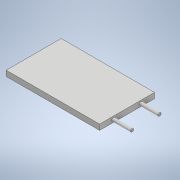
# Autodesk Inventor part: top
Saved by Autodesk Inventor 2022 (Build 260153000, 153)
## iProperties
Created: 2021-12-07
Part Number: top
Material: Generic
Document SubType Name: Modeling
Designer: cs1190490
Density: 1 g/cm^3
Appearance: Default
Author: cs1190490
Autodesk Inventor part; units mm, degrees
ref_plane "YZ Plane" through (0, 0, 0) normal (1, 0, 0) x (0, 1, 0)
ref_plane "XZ Plane" through (0, 0, 0) normal (0, 1, 0) x (-1, 0, 0)
ref_plane "XY Plane" through (0, 0, 0) normal (0, 0, 1) x (1, 0, 0)
sketch "Sketch1" plane through (0, 0, 0) normal (0, 0, 1) x (1, 0, 0)
  line L0 (-850, -500) -> (850, -500)
  line L1 (850, -500) -> (850, 500)
  line L2 (850, 500) -> (-850, 500)
  line L3 (-850, 500) -> (-850, -500)
  line L4 (-850, -500) -> (850, 500) construction
  line L5 (850, -500) -> (-850, 500) construction
  point P0 (0, 0)
  dimension "d0" = 1700
  dimension "d1" = 1000
  constraints: 12 end point, 2 midpoint, 2 parallel, 1 horizontal, 1 perpendicular
  measures "d0" distance of L1.end L2.end
  measures "d1" distance of L2.end L0.start
extrude "Extrusion1" add sketch "Sketch1" along normal blind 100
sketch "Sketch2" plane through (0, 0, 0) normal (0, 0, -1) x (-1, 0, 0)
  line L0 (-817.5, 467.5) -> (817.5, 467.5)
  line L1 (817.5, 467.5) -> (817.5, -467.5)
  line L2 (817.5, -467.5) -> (-817.5, -467.5)
  line L3 (-817.5, -467.5) -> (-817.5, 467.5)
  line L4 (-817.5, 467.5) -> (817.5, -467.5) construction
  line L5 (817.5, 467.5) -> (-817.5, -467.5) construction
  line L6 (850, 500) -> (850, -500) projected
  line L7 (850, -500) -> (-850, -500) projected
  point P0 (0, 0)
  dimension "d4" = 32.5
  dimension "d5" = 32.5
  constraints: 12 end point, 2 midpoint, 2 parallel, 1 horizontal, 1 perpendicular
  measures "d4" distance between parallel lines of L6 L1
  measures "d5" distance between parallel lines of L7 L2
extrude "Extrusion2" cut sketch "Sketch2" against normal blind 60
sketch "Sketch3" plane through (850, -500, 0) normal (1, 0, 0) x (0, 0, -1)
  circle A0 centre (-50, 250) radius 30
  circle A1 centre (-50, 750) radius 30
  point P0 (0, 500)
  dimension "d8" = 60
  dimension "d9" = 60
  constraints: 2 centre point
  measures "d8" diameter of A0
  measures "d9" diameter of A1
extrude "Extrusion3" add sketch "Sketch3" along normal blind 350 contours A0
sketch "Sketch4" plane through (850, -500, 0) normal (1, 0, 0) x (0, 0, -1)
  circle A0 centre (-50, 750) radius 30
  point P0 (0, 500)
  dimension "d12" = 60
  constraints: 1 centre point
  measures "d12" diameter of A0
extrude "Extrusion4" add sketch "Sketch4" along normal blind 350
chamfer "Chamfer1" distance 10 angle 45 1 edges at (1200, -250, 80)
chamfer "Chamfer2" distance 10 angle 45 1 edges at (1200, 250, 80)
body "Solid1"
